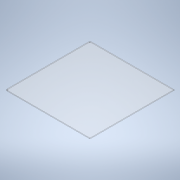
# Autodesk Inventor part: Wall_Back_ext
Saved by Autodesk Inventor 2020 (Build 240168000, 168)
## iProperties
Created: 2020-05-07
Part Number: Wall_Back_ext
Material: Типовые
Document SubType Name: Modeling
Designer: Михаил
Density: 1 g/cm^3
Appearance: По умолчанию
Author: Михаил
Autodesk Inventor part; units mm, degrees
ref_plane "YZ Plane" through (0, 0, 0) normal (1, 0, 0) x (0, 1, 0)
ref_plane "XZ Plane" through (0, 0, 0) normal (0, 1, 0) x (-1, 0, 0)
ref_plane "XY Plane" through (0, 0, 0) normal (0, 0, 1) x (1, 0, 0)
sketch "Эскиз1" plane through (0, 0, 0) normal (0, 1, 0) x (-1, 0, 0)
  line L0 (0, -408) -> (0, 0)
  line L1 (408, -4) -> (404, -4)
  line L2 (404, -4) -> (404, 0)
  line L3 (404, 0) -> (0, 0)
  line L4 (404, -408) -> (404, -404)
  line L5 (408, -404) -> (404, -404)
  line L6 (408, -4) -> (408, -404)
  line L7 (404, -408) -> (0, -408)
  dimension "d4" = 4
  dimension "d5" = 4
  dimension "d8" = 404
  dimension "d10" = 400
  dimension "d13" = 408
  dimension "d15" = 4
  dimension "d16" = 4
  constraints: 16 end point, 4 perpendicular, 2 horizontal
  measures "d4" distance of L1.start L1.end
  measures "d5" distance of L1.end L2.end
  measures "d8" distance of L4.start L0.start
  measures "d10" distance of L1.start L5.start
  measures "d13" distance from line of L7 L0.end
  measures "d15" distance between parallel lines of L5 L7
  measures "d16" distance of L5.start L4.end
extrude "Выдавливание1" add sketch "Эскиз1" along normal blind 4
